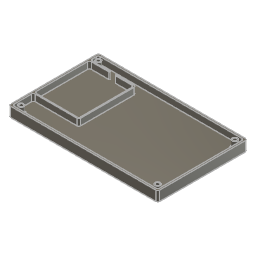
Bottom Case (Battery Tray) v13 (Autodesk Fusion 360 design; units mm, degrees)
Autodesk Fusion 360 part; units mm, degrees
sketch "Sketch1" plane through (0, 0, 0) normal (0, 1, 0) x (1, 0, 0)
  line L0 (0, 0) -> (162, 0) construction
  line L1 (162, 0) -> (162, 95) construction
  line L2 (162, 95) -> (0, 95) construction
  line L3 (0, 95) -> (0, 0) construction
  line L4 (4, 91) -> (158, 91) construction
  line L5 (158, 91) -> (158, 4) construction
  line L6 (158, 4) -> (4, 4) construction
  line L7 (4, 4) -> (4, 91) construction
  circle A0 centre (4, 91) radius 2
  circle A1 centre (4, 4) radius 2
  circle A2 centre (158, 4) radius 2
  circle A3 centre (158, 91) radius 2
  line L8 (-1, 96) -> (163, 96)
  line L9 (163, 96) -> (163, -1)
  line L10 (163, -1) -> (-1, -1)
  line L11 (-1, -1) -> (-1, 96)
  line L12 (4, 91) -> (158, 4) construction
  line L13 (162, 95) -> (0, 0) construction
  dimension "d1" = 162
  dimension "d2" = 95
  dimension "d7" = 4
  dimension "d8" = 1
  dimension "d9" = 1
  dimension "d10" = 1
  dimension "d11" = 1
  dimension "d55" = 87
  dimension "d56" = 154
  constraint horizontal L0
  constraint vertical L1
  constraint horizontal L2
  constraint vertical L3
  constraint coincident L0.start L3.end
  constraint horizontal L4
  constraint vertical L5
  constraint horizontal L6
  constraint vertical L7
  constraint coincident L4.start L7.end
  constraint coincident L6.end L7.start
  constraint coincident L5.end L6.start
  constraint coincident L4.end L5.start
  constraint equal A0 A1
  constraint equal A1 A2
  constraint equal A2 A3
  constraint horizontal L8
  constraint vertical L9
  constraint horizontal L10
  constraint vertical L11
  constraint midpoint L12 L13
  measures "d1" distance of L1.end L2.end
  measures "d2" distance of L0.start L2.end
  measures "d7" diameter of A0
  measures "d8" distance of L2 L8
  measures "d9" distance of L3 L11
  measures "d10" distance of L0 L10
  measures "d11" distance of L1 L9
  measures "d55" distance of L4.start L6.end
  measures "d56" distance of L4.start L4.end
extrude "Extrude1" add sketch "Sketch1" along normal blind 3
sketch "Sketch2" plane through (0, 0, 0) normal (0, -1, 0) x (1, 0, 0)
  circle A0 centre (4, -91) radius 2
  circle A1 centre (158, -4) radius 2
  circle A2 centre (4, -4) radius 2
  circle A3 centre (158, -91) radius 2
  line L0 (163, 1) -> (-1, 1)
  line L1 (-1, 1) -> (-1, -96)
  line L2 (-1, -96) -> (163, -96)
  line L3 (163, -96) -> (163, 1)
  line L4 (-3, 3) -> (165, 3)
  line L5 (165, 3) -> (165, -98)
  line L6 (165, -98) -> (-3, -98)
  line L7 (-3, -98) -> (-3, 3)
  dimension "d16" = 2
  dimension "d17" = 2
  dimension "d18" = 2
  dimension "d19" = 2
  constraint horizontal L4
  constraint vertical L5
  constraint horizontal L6
  constraint vertical L7
  measures "d16" distance of L0 L4
  measures "d17" distance of L2 L6
  measures "d18" distance of L1 L7
  measures "d19" distance of L3 L5
extrude "Extrude2" add sketch "Sketch2" against normal blind 9 contours L4 L5 L6 L7
fillet "Fillet2" radius 2 4 edges at (-3, 4.5, 3) (-3, 4.5, -98) (165, 4.5, -98) (165, 4.5, 3)
sketch "Sketch3" plane through (0, 3, 0) normal (0, 1, 0) x (-1, 0, 0)
  circle A0 centre (-4, -91) radius 2
  circle A1 centre (-158, -4) radius 2
  circle A2 centre (-4, -4) radius 2
  circle A3 centre (-158, -91) radius 2
  line L0 (1, 1) -> (-163, 1)
  line L1 (-163, 1) -> (-163, -96)
  line L2 (-163, -96) -> (1, -96)
  line L3 (1, -96) -> (1, 1)
  line L4 (1, -86) -> (-49, -86)
  line L5 (-49, -86) -> (-49, -24)
  line L6 (-49, -24) -> (1, -24)
  line L7 (1, -24) -> (1, -86)
  line L8 (1, -87.2) -> (-50.2, -87.2)
  line L9 (-50.2, -87.2) -> (-50.2, -22.8)
  line L10 (-50.2, -22.8) -> (1, -22.8)
  point P0 (-24, -86)
  dimension "d24" = 50
  dimension "d25" = 62
  dimension "d26" = 10
  dimension "d28" = 1.2
  dimension "d29" = 1.2
  dimension "d30" = 1.2
  constraint horizontal L4
  constraint vertical L5
  constraint horizontal L6
  constraint vertical L7
  constraint midpoint L4 P0
  constraint coincident L3 L4.start
  constraint coincident L3 L8.start
  constraint perpendicular L3 L8
  constraint perpendicular L8 L9
  constraint coincident L3 L10.end
  constraint perpendicular L3 L10
  measures "d24" distance of L4.start L4.end
  measures "d25" distance of L4.end L5.end
  measures "d26" distance of L2 L4
  measures "d28" distance of L4 L8
  measures "d29" distance of L5 L9
  measures "d30" distance of L6 L10
extrude "Extrude3" add sketch "Sketch3" along normal up to surface (6 mm away) contours L3 L4 L5 L6 L8 L9 L10
fillet "Fillet3" radius 2 4 edges at (-1, 6, -22.8) (50.2, 6, -22.8) (50.2, 6, -87.2) (-1, 6, -87.2)
sketch "Sketch4" plane through (0, 9, 0) normal (0, 1, 0) x (-1, 0, 0)
  arc A0 (-50.2, -85.2) -> (-48.2, -87.2) centre (-48.2, -85.2) ccw
  line L0 (-48.2, -87.2) -> (-1, -87.2)
  arc A1 (1, -89.2) -> (-1, -87.2) centre (-1, -89.2) ccw
  line L1 (1, -89.2) -> (1, -96)
  line L2 (1, -96) -> (-163, -96)
  line L3 (-163, -96) -> (-163, 1)
  line L4 (-163, 1) -> (1, 1)
  line L5 (1, 1) -> (1, -20.8)
  arc A2 (-1, -22.8) -> (1, -20.8) centre (-1, -20.8) ccw
  line L6 (-1, -22.8) -> (-48.2, -22.8)
  arc A3 (-48.2, -22.8) -> (-50.2, -24.8) centre (-48.2, -24.8) ccw
  line L7 (-50.2, -24.8) -> (-50.2, -85.2)
  arc A4 (-163, 3) -> (-165, 1) centre (-163, 1) ccw
  line L8 (-165, 1) -> (-165, -96)
  arc A5 (-165, -96) -> (-163, -98) centre (-163, -96) ccw
  line L9 (-163, -98) -> (1, -98)
  arc A6 (1, -98) -> (3, -96) centre (1, -96) ccw
  line L10 (3, -96) -> (3, 1)
  arc A7 (3, 1) -> (1, 3) centre (1, 1) ccw
  line L11 (1, 3) -> (-163, 3)
  line L12 (1, -86) -> (-49, -86)
  line L13 (-49, -86) -> (-49, -24)
  line L14 (-49, -24) -> (1, -24)
  line L15 (1, -24) -> (1, -86)
  line L16 (-21.6, -87.2) -> (-27.6, -87.2)
  line L17 (-27.6, -87.2) -> (-27.6, -86)
  line L18 (-27.6, -86) -> (-21.6, -86)
  line L19 (-21.6, -86) -> (-21.6, -87.2)
  point P0 (-162.5, 1)
  point P1 (-162.5, -96)
  point P2 (1, -96)
  point P3 (1, 1)
  point P4 (-162, 0)
  point P5 (-162, -95)
  point P6 (0, -95)
  dimension "d35" = 6
  constraint horizontal L16
  constraint vertical L17
  constraint horizontal L18
  constraint vertical L19
  constraint coincident L12 L17.end
  constraint coincident L0 L16.start
  constraint midpoint L0 L16
  measures "d35" distance of L16.start L16.end
extrude "Extrude4" cut sketch "Sketch4" against normal up to surface (6 mm away) contours L0 L12 L16 L17 L18 L19
fillet "Fillet4" radius 2 4 edges at (-1, 6, -86) (49, 6, -86) (49, 6, -24) (-1, 6, -24)
fillet "Fillet5" radius 2 4 edges at (-1, 6, -96) (163, 6, -96) (163, 6, 1) (-1, 6, 1)
fillet "Fillet6" radius 0.6 4 edges at (21.6, 6, -86) (21.6, 6, -87.2) (27.6, 6, -86) (27.6, 6, -87.2)
sketch "Sketch5" plane through (0, 3, 0) normal (0, 1, 0) x (-1, 0, 0)
  circle A0 centre (-4, -91) radius 2
  circle A1 centre (-158, -4) radius 2
  circle A2 centre (-4, -4) radius 2
  circle A3 centre (-158, -91) radius 2
  arc A4 (1, -1) -> (-1, 1) centre (-1, -1) ccw
  line L0 (-1, 1) -> (-161, 1)
  arc A5 (-161, 1) -> (-163, -1) centre (-161, -1) ccw
  line L1 (-163, -1) -> (-163, -94)
  arc A6 (-163, -94) -> (-161, -96) centre (-161, -94) ccw
  line L2 (-161, -96) -> (-1, -96)
  arc A7 (-1, -96) -> (1, -94) centre (-1, -94) ccw
  line L3 (1, -94) -> (1, -89.2)
  arc A8 (1, -89.2) -> (-1, -87.2) centre (-1, -89.2) ccw
  line L4 (-1, -87.2) -> (-21, -87.2)
  arc A9 (-21, -86) -> (-21, -87.2) centre (-21, -86.6) ccw
  line L5 (-21, -86) -> (-1, -86)
  arc A10 (-1, -86) -> (1, -84) centre (-1, -84) ccw
  line L6 (1, -84) -> (1, -26)
  arc A11 (1, -26) -> (-1, -24) centre (-1, -26) ccw
  line L7 (-1, -24) -> (-47, -24)
  arc A12 (-47, -24) -> (-49, -26) centre (-47, -26) ccw
  line L8 (-49, -26) -> (-49, -84)
  arc A13 (-49, -84) -> (-47, -86) centre (-47, -84) ccw
  line L9 (-47, -86) -> (-28.2, -86)
  arc A14 (-28.2, -87.2) -> (-28.2, -86) centre (-28.2, -86.6) ccw
  line L10 (-28.2, -87.2) -> (-48.2, -87.2)
  arc A15 (-50.2, -85.2) -> (-48.2, -87.2) centre (-48.2, -85.2) ccw
  line L11 (-50.2, -85.2) -> (-50.2, -24.8)
  arc A16 (-48.2, -22.8) -> (-50.2, -24.8) centre (-48.2, -24.8) ccw
  line L12 (-48.2, -22.8) -> (-1, -22.8)
  arc A17 (-1, -22.8) -> (1, -20.8) centre (-1, -20.8) ccw
  line L13 (1, -20.8) -> (1, -1)
  circle A18 centre (-4, -91) radius 3
  circle A19 centre (-158, -91) radius 3
  circle A20 centre (-158, -4) radius 3
  circle A21 centre (-4, -4) radius 3
  dimension "d44" = 6
  constraint concentric A0 A18
  constraint concentric A3 A19
  constraint concentric A1 A20
  constraint concentric A2 A21
  constraint equal A18 A21
  constraint equal A18 A19
  constraint equal A19 A20
  measures "d44" diameter of A18
extrude "Extrude5" add sketch "Sketch5" along normal up to surface (7.5 mm away) contours A18 | A19 | A20 | A21
fillet "Fillet7" radius 1 4 edges at (6.797, 3, -2.9152) (6.797, 3, -89.9152) (160.797, 3, -89.9152) (160.797, 3, -2.9152)
extrude "Extrude6" add 1 faces at (106.0424, 0, -61.6396) along direction (0, -1, 0) blind 0.6
sketch "Sketch6" plane through (0, -0.6, 0) normal (0, -1, 0) x (1, 0, 0)
  arc A0 (165, 1) -> (163, 3) centre (163, 1) ccw
  line L0 (163, 3) -> (-1, 3)
  arc A1 (-1, 3) -> (-3, 1) centre (-1, 1) ccw
  line L1 (-3, 1) -> (-3, -96)
  arc A2 (-3, -96) -> (-1, -98) centre (-1, -96) ccw
  line L2 (-1, -98) -> (163, -98)
  arc A3 (163, -98) -> (165, -96) centre (163, -96) ccw
  line L3 (165, -96) -> (165, 1)
  circle A4 centre (4, -91) radius 2
  circle A5 centre (158, -4) radius 2
  circle A6 centre (4, -4) radius 2
  circle A7 centre (158, -91) radius 2
  circle A8 centre (4, -4) radius 4
  circle A9 centre (158, -4) radius 4
  circle A10 centre (158, -91) radius 4
  circle A11 centre (4, -91) radius 4
  dimension "d51" = 8
  constraint concentric A6 A8
  constraint concentric A5 A9
  constraint concentric A7 A10
  constraint concentric A4 A11
  constraint equal A8 A9
  constraint equal A9 A10
  constraint equal A10 A11
  measures "d51" diameter of A8
extrude "Extrude7" cut sketch "Sketch6" against normal blind 3 contours A8 | A9 | A10 | A11
extrude "Extrude8" add 1 faces at (-2.3333, 9, -40.3333) along direction (0, 1, 0) blind 1.5
